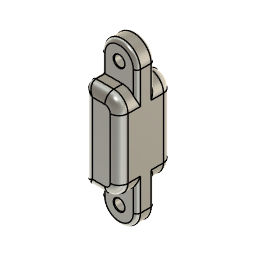
middle v1 (Autodesk Fusion 360 design; units mm, degrees)
Autodesk Fusion 360 part; units mm, degrees
sketch "Çizim1" plane through (0, 0, 0) normal (0, 1, 0) x (1, 0, 0)
  circle A0 centre (0, 0) radius 10
  dimension "d1" = 20
  constraint coincident A0.centre origin
  measures "d1" diameter of A0
extrude "Ekstrüzyon1" add sketch "Çizim1" along normal blind 10
sketch "Çizim2" plane through (0, 0, 0) normal (0, -1, 0) x (1, 0, 0)
  circle A0 centre (0, 0) radius 10
  line L0 (-10, 0) -> (10, 0)
  line L1 (10, 0) -> (10, -80)
  line L2 (10, -80) -> (-10, -80)
  line L3 (-10, -80) -> (-10, 0)
  dimension "d4" = 80
  constraint horizontal L0
  constraint vertical L1
  constraint horizontal L2
  constraint vertical L3
  constraint coincident A0 L0.start
  measures "d4" distance of L0.start L2.end
extrude "Ekstrüzyon2" add sketch "Çizim2" against normal blind 10 contours A0 L1 L2 L3
sketch "Çizim3" plane through (0, 0, 0) normal (0, -1, 0) x (1, 0, 0)
  arc A0 (10, 0) -> (-10, 0) centre (0, 0) ccw
  line L0 (-10, 0) -> (-10, -80)
  line L1 (-10, -80) -> (10, -80)
  line L2 (10, -80) -> (10, 0)
  line L3 (-10, -10) -> (10, -10)
  line L4 (10, -10) -> (10, -60)
  line L5 (10, -60) -> (-10, -60)
  line L6 (-10, -60) -> (-10, -10)
  dimension "d7" = 20
  dimension "d8" = 50
  constraint horizontal L3
  constraint vertical L4
  constraint horizontal L5
  constraint vertical L6
  constraint coincident L0 L3.start
  measures "d7" distance of L3.start L3.end
  measures "d8" distance of L3.start L5.end
extrude "Ekstrüzyon3" add sketch "Çizim3" along normal blind 10 contours L0 L2 L3 L4 L5 L6
sketch "Çizim4" plane through (0, 10, 0) normal (0, 1, 0) x (-1, 0, 0)
  arc A0 (10, 0) -> (-10, 0) centre (0, 0) ccw
  line L0 (-10, 0) -> (-10, -80)
  line L1 (-10, -80) -> (10, -80)
  line L2 (10, -80) -> (10, 0)
  line L3 (-10, -10) -> (10, -10)
  line L4 (10, -10) -> (10, -60)
  line L5 (10, -60) -> (-10, -60)
  line L6 (-10, -60) -> (-10, -10)
  dimension "d11" = 50
  constraint horizontal L3
  constraint vertical L4
  constraint horizontal L5
  constraint vertical L6
  constraint coincident L0 L3.start
  measures "d11" distance of L3.start L5.end
extrude "Ekstrüzyon4" add sketch "Çizim4" along normal blind 10 contours L0 L2 L3 L4 L5 L6
sketch "Çizim5" plane through (0, 0, 0) normal (0, -1, 0) x (1, 0, 0)
  line L0 (10, -60) -> (-10, -60)
  line L1 (-10, -60) -> (-10, -80)
  line L2 (-10, -80) -> (10, -80)
  line L3 (10, -80) -> (10, -60)
  circle A0 centre (0, -70) radius 10
  dimension "d14" = 20
  measures "d14" diameter of A0
extrude "Ekstrüzyon5" cut sketch "Çizim5" against normal blind 15 contours L2 L3 A0 | L1 L2 A0
sketch "Çizim6" plane through (0, 10, 0) normal (0, 1, 0) x (-1, 0, 0)
  line L0 (-10, -10) -> (10, -10)
  line L1 (10, -10) -> (10, 0)
  arc A0 (10, 0) -> (-10, 0) centre (0, 0) ccw
  line L2 (-10, 0) -> (-10, -10)
  circle A1 centre (0, 0) radius 3
  dimension "d17" = 6
  constraint coincident A0.centre A1.centre
  measures "d17" diameter of A1
extrude "Ekstrüzyon6" cut sketch "Çizim6" against normal blind 105 contours A1
sketch "Çizim7" plane through (0, 10, 0) normal (0, 1, 0) x (-1, 0, 0)
  arc A0 (-10, -70) -> (10, -70) centre (0, -70) ccw
  line L0 (10, -70) -> (10, -60)
  line L1 (10, -60) -> (-10, -60)
  line L2 (-10, -60) -> (-10, -70)
  circle A1 centre (0, -70) radius 3
  dimension "d20" = 6
  constraint concentric A0 A1
  measures "d20" diameter of A1
extrude "Ekstrüzyon7" cut sketch "Çizim7" against normal blind 34 contours A1
fillet "Radyus1" radius 2 12 edges at (-10, 0, -5) (0, 0, 10) (10, 0, -5) (-10, 10, -5) (0, 10, 10) (10, 10, -5) (10, 0, -65) (0, 0, -80) (-10, 0, -65) (10, 10, -65) (0, 10, -80) (-10, 10, -65)
fillet "Radyus2" radius 5 2 faces at (-3.3333, -10, -43.3333) (3.3333, 20, -43.3333)
fillet "Radyus3" radius 0.3 4 edges at (2.797, 0, -1.0848) (2.797, 10, 1.0848) (2.797, 0, -71.0848) (2.797, 10, -68.9152)
fillet "Radyus4" radius 8 8 edges at (10, -1.5, -10) (8.5355, -8.5355, -11.4645) (10, 11.5, -10) (8.5355, 18.5355, -11.4645) (10, -1.5, -60) (8.5355, -8.5355, -58.5355) (10, 11.5, -60) (8.5355, 18.5355, -58.5355)
fillet "Radyus5" radius 2 8 edges at (-10, 11.5, -10) (-8.5355, 18.5355, -11.4645) (-10, -1.5, -10) (-8.5355, -8.5355, -11.4645) (-10, 11.5, -60) (-8.5355, 18.5355, -58.5355) (-10, -1.5, -60) (-8.5355, -8.5355, -58.5355)
